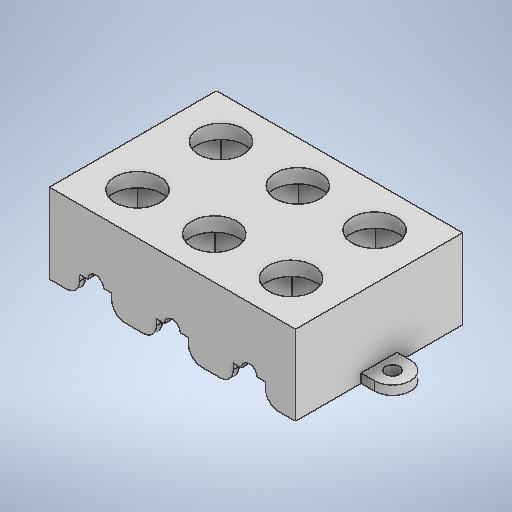
# Autodesk Inventor part: inner_top
Saved by Autodesk Inventor 2025.1 (Build 291241000, 241)
## iProperties
Created: 2025-02-27
Part Number: inner_top
Material: Generic
Document SubType Name: Modeling
Designer: santiago
Density: 1 g/cm^3
Appearance: Default
Author: santiago
Autodesk Inventor part; units mm, degrees
ref_plane "YZ Plane" through (0, 0, 0) normal (1, 0, 0) x (0, 1, 0)
ref_plane "XZ Plane" through (0, 0, 0) normal (0, 1, 0) x (-1, 0, 0)
ref_plane "XY Plane" through (0, 0, 0) normal (0, 0, 1) x (1, 0, 0)
sketch "Sketch1" plane through (0, 0, 0) normal (0, 1, 0) x (-1, 0, 0)
  line L0 (-8, 8) -> (8, 8)
  line L1 (8, 8) -> (8, -8)
  line L2 (8, -8) -> (-8, -8)
  line L3 (-8, -8) -> (-8, 8)
  line L4 (-8, 8) -> (8, -8) construction
  line L5 (8, 8) -> (-8, -8) construction
  line L6 (-9.3, 9.3) -> (9.3, 9.3)
  line L7 (9.3, 9.3) -> (9.3, -9.3)
  line L8 (9.3, -9.3) -> (-9.3, -9.3)
  line L9 (-9.3, -9.3) -> (-9.3, 9.3)
  line L10 (-9.3, 9.3) -> (9.3, -9.3) construction
  line L11 (9.3, 9.3) -> (-9.3, -9.3) construction
  point P0 (0, 0)
  dimension "d0" = 16
  dimension "d1" = 16
  dimension "d2" = 18.6
  dimension "d3" = 18.6
  constraints: 24 end point, 4 midpoint, 4 parallel, 2 horizontal, 2 perpendicular, 1 point on line
  measures "d0" distance of L1.end L2.end
  measures "d1" distance of L0.end L1.end
  measures "d2" distance of L7.end L8.end
  measures "d3" distance of L6.end L7.end
extrude "Extrusion1" add sketch "Sketch1" along normal blind 24
sketch "Sketch2" plane through (-9.3, 0, 9.3) normal (0, 0, 1) x (1, 0, 0)
  line L0 (18.6, 0) -> (0, 0) projected
  line L1 (5.55, 0) -> (13.05, 0)
  line L2 (13.05, 0) -> (13.05, 4.5)
  line L3 (13.05, 4.5) -> (5.55, 4.5)
  line L4 (5.55, 4.5) -> (5.55, 0)
  circle A0 centre (9.3, 4.5) radius 1.7375
  point P0 (9.3, 0)
  point P1 (9.3, 0)
  point P2 (13.05, 0)
  point P3 (11.0375, 4.5)
  point P4 (7.5625, 4.5)
  dimension "d6" = 7.5
  dimension "d7" = 4.5
  dimension "d11" = 3.475
  constraints: 8 end point, 2 midpoint, 2 parallel, 1 centre point, 1 coincident, 1 horizontal, 1 perpendicular, 1 point on line, 1 vertical alignment
  measures "d6" distance of L3.end L2.end
  measures "d7" distance of L1.end L2.end
  measures "d11" diameter of A0
extrude "Extrusion2" cut sketch "Sketch2" against normal through all
fillet "Fillet1" radius 3.3 4 edges at (-3.75, 0, -8.65) (-3.75, 0, 8.65) (3.75, 0, 8.65) (3.75, 0, -8.65)
sketch "Sketch4" plane through (0, 24, 0) normal (0, 1, 0) x (1, 0, 0)
  line L0 (7.05, 8) -> (8, 8) projected
  line L1 (-7.05, -8) -> (-8, -8) projected
  line L2 (8, 8) -> (-8, 8)
  line L3 (-8, 8) -> (-8, -8)
  line L4 (-8, -8) -> (8, -8)
  line L5 (8, -8) -> (8, 8)
  point P0 (0, 0)
  constraints: 8 end point, 2 parallel, 1 horizontal, 1 perpendicular
extrude "Extrusion3" add sketch "Sketch4" against normal blind 8
sketch "Sketch5" plane through (0, 24, 0) normal (0, 1, 0) x (1, 0, 0)
  circle A0 centre (0, 0) radius 5.25
  dimension "d14" = 10.5
  constraints: 1 centre point, 1 coincident
  measures "d14" diameter of A0
sketch "Sketch6" plane through (0, 16, 0) normal (0, -1, 0) x (1, 0, 0)
  circle A0 centre (0, 0) radius 5.9
  dimension "d15" = 11.8
  constraints: 1 centre point, 1 coincident
  measures "d15" diameter of A0
loft "Loft1" cut profiles "Sketch6", "Sketch5"
fillet "Fillet2" radius 0.5 2 edges at (-5.25, 24, 0) (-5.9, 16, 0)
pattern_linear "Rectangular Pattern2" count 2 spacing 18.6 along (0, 0, 1) count 3 spacing 17.1 along (-1, 0, 0)
sketch "Sketch7" plane through (0, 0, 0) normal (0, -1, 0) x (1, 0, 0)
  circle A0 centre (13.3, 9.3) radius 2.75
  circle A1 centre (-47.5, 9.3) radius 2.75
  line L0 (9.3, 27.9) -> (9.3, -9.3) projected
  line L1 (-43.5, -9.3) -> (-43.5, 27.9) projected
  circle A2 centre (13.3, 9.3) radius 4
  circle A3 centre (-47.5, 9.3) radius 4
  line L2 (-47.5, 13.3) -> (-43.5, 13.3)
  line L3 (-47.5, 5.3) -> (-43.5, 5.3)
  line L4 (13.3, 5.3) -> (9.3, 5.3)
  line L5 (13.3, 13.3) -> (9.3, 13.3)
  point P0 (0, 0)
  point P1 (9.3, 9.3)
  point P2 (-43.5, 9.3)
  dimension "d33" = 5.5
  dimension "d34" = 5.5
  dimension "d35" = 4
  dimension "d36" = 4
  constraints: 8 end point, 8 point on line, 6 point on circle, 4 centre point, 2 coincident, 2 midpoint, 2 perpendicular, 2 tangent
  measures "d33" diameter of A0
  measures "d34" diameter of A1
  measures "d35" distance of A2.start A0.centre
  measures "d36" distance of A3.start A1.centre
extrude "Extrusion4" add sketch "Sketch7" along normal blind 27.8 and the other way blind 6
sketch "Sketch8" plane through (0, -27.8, 0) normal (0, -1, 0) x (1, 0, 0)
  circle A0 centre (13.3, 9.3) radius 2.75 projected
  circle A1 centre (13.3, 9.3) radius 1.6
  circle A2 centre (-47.5, 9.3) radius 2.75 projected
  circle A3 centre (-47.5, 9.3) radius 1.6
  circle A4 centre (-47.5, 9.3) radius 2.75 projected
  point P0 (0, 0)
  dimension "d41" = 3.2
  dimension "d42" = 3.2
  constraints: 2 centre point, 2 coincident
  measures "d41" diameter of A1
  measures "d42" diameter of A3
extrude "Extrusion5" add sketch "Sketch8" against normal blind 2
fillet "Fillet3" radius 3 4 edges at (9.3, 3, 13.3) (9.3, 3, 5.3) (-43.5, 3, 5.3) (-43.5, 3, 13.3)
fillet "Fillet4" radius 2 6 edges at (-43.5, 6, 3.8) (-43.5, 6, 9.3) (-43.5, 6, 14.8) (9.3, 6, 14.8) (9.3, 6, 9.3) (9.3, 6, 3.8)
equation "\"d33\" = d34"
body "Solid1"
